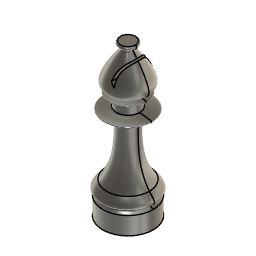
bishop (Autodesk Fusion 360 design; units mm, degrees)
Autodesk Fusion 360 part; units mm, degrees
note: some values were not read from the file. Set by a fixed rule: which sketch regions a step uses.
sketch "Profile" plane through (0, 0, 0) normal (0, 1, 0) x (1, 0, 0)
  line L0 (4.127, 0) -> (12.7, 0)
  line L1 (0, -8.1) -> (0, -76.2)
  line L2 (4.127, -8.1) -> (4.127, 0)
  line L3 (4.127, -8.1) -> (0, -8.1)
  line L4 (12.7, 0) -> (12.7, -8.89)
  spline S0 degree 5 poles (5.143, -41.873) (5.1376, -42.1632) (5.1518, -42.7019) (5.2475, -43.3847) (5.5006, -44.0552) (5.903, -44.5571) (6.2607, -44.8097) (6.4898, -44.9091) (6.6093, -44.9474) (6.7976, -44.999) (7.2823, -45.1181) (8.2252, -45.3358) (9.6189, -45.6575) (11.1517, -46.0576) (12.1723, -46.4811) (12.1726, -46.8681) (10.9092, -47.1683) (9.2364, -47.371) (8.0799, -47.497) (7.4832, -47.5696) (7.2335, -47.6184) (6.9523, -47.6595) (6.5113, -47.7007) (6.0868, -47.7339) (5.842, -47.752) knots 0 0 0 0 0 0 0.05 0.1 0.15 0.2 0.25 0.3 0.35 0.4 0.45 0.5 0.55 0.6 0.65 0.7 0.75 0.8 0.85 0.9 0.95 1 1 1 1 1 1
  line L5 (5.1918, -39.2405) -> (5.0943, -44.5054)
  line L6 (12.8124, -46.7744) -> (8.89, -47.498)
  line L7 (7.6704, -47.6171) -> (4.0136, -47.8869)
  spline S1 degree 5 poles (10.7494, -15.8342) (10.521, -16.1371) (10.076, -16.7523) (9.4443, -17.7034) (8.6738, -19.0284) (7.833, -20.7802) (7.1175, -22.6259) (6.5283, -24.5581) (6.0629, -26.5614) (5.7123, -28.6072) (5.4613, -30.6559) (5.2919, -32.663) (5.1854, -34.5837) (5.1248, -36.3781) (5.0964, -38.0171) (5.0918, -39.4878) (5.1035, -40.5268) (5.1202, -41.2295) (5.1348, -41.6641) (5.143, -41.873) knots 0 0 0 0 0 0 0.066667 0.133333 0.2 0.266667 0.333333 0.4 0.466667 0.533333 0.6 0.666667 0.733333 0.8 0.866667 0.933333 1 1 1 1 1 1
  spline S2 degree 5 poles (5.842, -53.1133) (5.8827, -53.127) (5.9672, -53.1543) (6.1031, -53.1948) (6.3026, -53.2476) (6.5824, -53.3121) (6.8912, -53.3753) (7.2263, -53.4378) (7.5823, -53.5008) (7.9511, -53.5659) (8.3211, -53.6347) (8.6761, -53.7087) (8.9953, -53.7891) (9.2521, -53.8764) (9.4141, -53.9699) (9.452, -54.0686) (9.3466, -54.171) (9.0984, -54.2754) (8.7256, -54.38) (8.258, -54.4833) (7.732, -54.5837) (7.1847, -54.6799) (6.6493, -54.7708) (6.1493, -54.8556) (5.6995, -54.934) (5.3084, -55.0058) (5.0456, -55.0579) (4.877, -55.0939) (4.7774, -55.1166) (4.7307, -55.1276) knots 0 0 0 0 0 0 0.04 0.08 0.12 0.16 0.2 0.24 0.28 0.32 0.36 0.4 0.44 0.48 0.52 0.56 0.6 0.64 0.68 0.72 0.76 0.8 0.84 0.88 0.92 0.96 1 1 1 1 1 1
  spline S3 degree 5 poles (3.81, -76.2) (3.8957, -76.1495) (4.0532, -76.0488) (4.248, -75.8987) (4.4245, -75.7001) (4.5084, -75.4542) (4.4612, -75.2089) (4.295, -74.9604) (4.0297, -74.7053) (3.6929, -74.4446) (3.3208, -74.1878) (2.9574, -73.9547) (2.6497, -73.7585) (2.4433, -73.5961) (2.3774, -73.4296) (2.4811, -73.1883) (2.7703, -72.798) (3.2439, -72.2088) (3.8844, -71.4029) (4.6619, -70.3861) (5.5367, -69.1847) (6.4629, -67.8398) (7.3911, -66.4029) (8.2716, -64.9313) (9.0576, -63.4831) (9.7083, -62.1129) (10.1915, -60.867) (10.4874, -59.7787) (10.5917, -58.8633) (10.5175, -58.115) (10.2895, -57.5141) (9.9402, -57.0323) (9.5049, -56.6385) (9.0174, -56.3042) (8.505, -56.0098) (7.9863, -55.7476) (7.4731, -55.5174) (6.9722, -55.3243) (6.4872, -55.1755) (6.0193, -55.0773) (5.5696, -55.0334) (5.2247, -55.0429) (4.9744, -55.0754) (4.8113, -55.1083) (4.7307, -55.1276) knots 0 0 0 0 0 0 0.025 0.05 0.075 0.1 0.125 0.15 0.175 0.2 0.225 0.25 0.275 0.3 0.325 0.35 0.375 0.4 0.425 0.45 0.475 0.5 0.525 0.55 0.575 0.6 0.625 0.65 0.675 0.7 0.725 0.75 0.775 0.8 0.825 0.85 0.875 0.9 0.925 0.95 0.975 1 1 1 1 1 1
  line L8 (5.842, -47.752) -> (5.842, -53.1133)
  spline S4 degree 5 poles (12.7, -8.89) (12.4864, -9.0092) (12.0953, -9.238) (11.6165, -9.5528) (11.1952, -9.9154) (11.0241, -10.276) (11.1812, -10.5549) (11.605, -10.7754) (12.1827, -10.9792) (12.7728, -11.218) (13.2359, -11.541) (13.4591, -11.985) (13.3914, -12.5609) (13.0421, -13.2541) (12.4598, -14.0341) (11.839, -14.7265) (11.3278, -15.2555) (10.9723, -15.6127) (10.7798, -15.804) (10.7494, -15.8342) knots 0 0 0 0 0 0 0.05 0.1 0.15 0.2 0.25 0.3 0.35 0.4 0.45 0.5 0.55 0.6 0.65 0.7 0.709382 0.709382 0.709382 0.709382 0.709382 0.709382
  line L9 (3.81, -76.2) -> (0, -76.2)
  point P0 (11.2931, -10.578)
  point P1 (13.2868, -11.7259)
  point P2 (10.8512, -47.1362)
  point P3 (9.2425, -45.5762)
  point P4 (6.4638, -44.8937)
  point P5 (8.6096, -46.99)
  point P6 (6.35, -25.4)
  point P7 (5.1371, -36.1843)
  point P8 (8.9323, -53.7773)
  point P9 (9.398, -54.102)
  point P10 (7.1253, -54.6894)
  point P11 (7.0726, -53.4086)
  point P12 (3.7646, -74.5055)
  point P13 (2.54, -73.66)
  point P14 (2.624, -73.0061)
  point P15 (10.3867, -60.0643)
  point P16 (9.1983, -56.4374)
  point P17 (6.6142, -55.2213)
  point P18 (4.4744, -75.3678)
  dimension "d1" = 12.7
  dimension "d2" = 76.2
  dimension "d5" = 8.89
  dimension "d9" = 4.127
  dimension "d10" = 8.1
  constraint horizontal L0
  constraint perpendicular L0 L1
  constraint perpendicular L0 L2
  constraint perpendicular L1 L3
  constraint perpendicular L0 L4
  constraint midpoint S0.start L5
  constraint midpoint P2 L6
  constraint midpoint S0.end L7
  constraint parallel L1 L8
  constraint coincident S1.start S4.end
  measures "d1" distance of origin L0.end
  measures "d2" distance of origin L1.end
  measures "d5" distance of L0.end L4.end
  measures "d9" distance of L1.start L2.start
  measures "d10" distance of L0.start L2.start
revolve "Revolve1" add sketch "Profile" angle 360 about axis through (0, 0, 8.1) along (0, 0, 1)
sketch "Slit" plane through (0, 0, 0) normal (0, 1, 0) x (1, 0, 0)
  spline S0 degree 5 poles (4.9108, -70.9064) (4.7639, -70.8022) (4.4757, -70.5899) (4.0601, -70.2589) (3.54, -69.7925) (2.9504, -69.1647) (2.4265, -68.4882) (1.9735, -67.7593) (1.5936, -66.9763) (1.2834, -66.1417) (1.0374, -65.2595) (0.8876, -64.519) (0.8, -63.9454) (0.7524, -63.5549) (0.7313, -63.3577) knots 0 0 0 0 0 0 0.1 0.2 0.3 0.4 0.5 0.6 0.7 0.8 0.9 1 1 1 1 1 1
  spline S1 degree 5 poles (5.334, -70.104) (5.1872, -69.9795) (4.9016, -69.7263) (4.4974, -69.3337) (4.0076, -68.784) (3.4827, -68.0507) (3.0525, -67.2671) (2.7242, -66.4294) (2.5006, -65.5362) (2.3761, -64.5904) (2.3428, -63.5963) (2.3829, -62.7656) (2.448, -62.1239) (2.5068, -61.688) (2.54, -61.468) knots 0 0 0 0 0 0 0.1 0.2 0.3 0.4 0.5 0.6 0.7 0.8 0.9 1 1 1 1 1 1
  line L0 (2.54, -61.468) -> (0.7313, -63.3577)
  line L1 (5.334, -70.104) -> (4.9108, -70.9064)
  point P0 (2.032, -67.818)
  point P1 (2.794, -66.548)
extrude "Extrude4" cut sketch "Slit" along normal blind 12.7 and the other way blind 12.7
